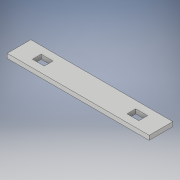
# Autodesk Inventor part: table_bottont
Saved by Autodesk Inventor 2019.4 (Build 234330000, 330)
## iProperties
Created: 2019-12-14
Part Number: table_bottont
Material: Generic
Document SubType Name: Modeling
Designer: fabfarm
Density: 1 g/cm^3
Appearance: Default
Author: fabfarm
Autodesk Inventor part; units mm, degrees
ref_plane "YZ Plane" through (0, 0, 0) normal (1, 0, 0) x (0, 1, 0)
ref_plane "XZ Plane" through (0, 0, 0) normal (0, 1, 0) x (-1, 0, 0)
ref_plane "XY Plane" through (0, 0, 0) normal (0, 0, 1) x (1, 0, 0)
sketch "Sketch1" plane through (0, 0, 0) normal (0, 0, 1) x (1, 0, 0)
  line L0 (0, 0) -> (600, 0)
  line L1 (600, 0) -> (600, 18.55)
  line L2 (600, 18.55) -> (0, 18.55)
  line L3 (0, 18.55) -> (0, 0)
  dimension "d0" = 600
  dimension "d1" = 18.55
  constraints: 8 end point, 2 parallel, 1 horizontal, 1 perpendicular
  measures "d0" distance of L1.end L2.end
  measures "d1" distance of L2.end L0.start
extrude "Extrusion1" add sketch "Sketch1" along normal blind 100
sketch "Sketch2" plane through (0, 18.55, 0) normal (0, 1, 0) x (1, 0, 0)
  line L0 (75, -31.45) -> (125, -31.45)
  line L1 (125, -31.45) -> (125, -68.55)
  line L2 (125, -68.55) -> (75, -68.55)
  line L3 (75, -68.55) -> (75, -31.45)
  line L4 (475, -31.45) -> (525, -31.45)
  line L5 (525, -31.45) -> (525, -68.55)
  line L6 (525, -68.55) -> (475, -68.55)
  line L7 (475, -68.55) -> (475, -31.45)
  line L8 (0, 0) -> (0, -100) projected
  line L9 (600, 0) -> (600, -100) projected
  line L10 (100, -31.45) -> (100, 0) construction
  line L11 (0, 0) -> (600, 0) projected
  line L12 (100, -68.55) -> (100, -100) construction
  line L13 (0, -100) -> (600, -100) projected
  dimension "d4" = 50
  dimension "d5" = 75
  dimension "d6" = 75
  dimension "d7" = 37.1
  dimension "d8" = 50
  constraints: 20 end point, 4 parallel, 4 point on line, 2 horizontal, 2 midpoint, 2 perpendicular, 2 vertical, 1 collinear
  measures "d4" distance of L0.start L0.end
  measures "d5" distance between parallel lines of L8 L3
  measures "d6" distance between parallel lines of L9 L5
  measures "d7" distance of L6.end L4.start
  measures "d8" distance between parallel lines of L5 L7
extrude "Extrusion2" cut sketch "Sketch2" against normal blind 100 contours L0 L1 L2 L3 | L4 L5 L6 L7
body "Solid1"
